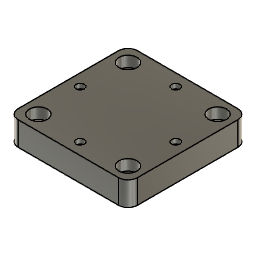
Base_North v3 (Autodesk Fusion 360 design; units mm, degrees)
Autodesk Fusion 360 part; units mm, degrees
note: some values were not read from the file. Set by a fixed rule: which sketch regions a step uses.
sketch "Sketch1" plane through (0, 0, 0) normal (0, 0, 1) x (1, 0, 0)
  line L0 (0, 0) -> (-50, 0)
  line L1 (-50, 0) -> (-50, 50)
  line L2 (-50, 50) -> (0, 50)
  line L3 (0, 50) -> (0, 0)
  dimension "d1" = 50
  dimension "d2" = 50
  constraint horizontal L0
  constraint vertical L1
  constraint horizontal L2
  constraint vertical L3
  constraint coincident L0.start L3.end
  measures "d1" distance of L0.start L0.end
  measures "d2" distance of L0.start L2.end
extrude "Extrude1" add sketch "Sketch1" along normal blind 10
sketch "Sketch2" plane through (0, 0, 10) normal (0, 0, 1) x (-1, 0, 0)
  line L0 (0, -50) -> (50, -50)
  line L1 (50, -50) -> (50, 0)
  line L2 (50, 0) -> (0, 0)
  line L3 (0, 0) -> (0, -50)
  line L4 (50, 0) -> (43.75, 0)
  line L5 (43.75, 0) -> (43.75, -6.25)
  line L6 (43.75, -6.25) -> (50, -6.25)
  line L7 (50, -6.25) -> (50, 0)
  line L8 (50, -50) -> (43.75, -50)
  line L9 (43.75, -50) -> (43.75, -43.75)
  line L10 (43.75, -43.75) -> (50, -43.75)
  line L11 (50, -43.75) -> (50, -50)
  line L12 (0, -50) -> (6.25, -50)
  line L13 (6.25, -50) -> (6.25, -43.75)
  line L14 (6.25, -43.75) -> (0, -43.75)
  line L15 (0, -43.75) -> (0, -50)
  line L16 (0, 0) -> (6.25, 0)
  line L17 (6.25, 0) -> (6.25, -6.25)
  line L18 (6.25, -6.25) -> (0, -6.25)
  line L19 (0, -6.25) -> (0, 0)
  circle A0 centre (43.75, -43.75) radius 3.75
  circle A1 centre (6.25, -43.75) radius 3.75
  circle A2 centre (43.75, -6.25) radius 3.75
  circle A3 centre (6.25, -6.25) radius 3.75
  dimension "d5" = 6.25
  dimension "d6" = 6.25
  dimension "d7" = 6.25
  dimension "d8" = 6.25
  dimension "d9" = 6.25
  dimension "d10" = 6.25
  dimension "d11" = 6.25
  dimension "d12" = 6.25
  dimension "d13" = 7.5
  dimension "d14" = 7.5
  dimension "d15" = 7.5
  dimension "d16" = 7.5
  constraint horizontal L4
  constraint vertical L5
  constraint horizontal L6
  constraint vertical L7
  constraint coincident L1.end L2.start
  constraint horizontal L8
  constraint vertical L9
  constraint horizontal L10
  constraint vertical L11
  constraint coincident L0.end L1.start
  constraint horizontal L12
  constraint vertical L13
  constraint horizontal L14
  constraint vertical L15
  constraint coincident L0.start L3.end
  constraint horizontal L16
  constraint vertical L17
  constraint horizontal L18
  constraint vertical L19
  constraint coincident L2.end L3.start
  constraint coincident L9.end L10.start
  constraint coincident L13.end L14.start
  constraint coincident L5.end L6.start
  constraint coincident L17.end L18.start
  measures "d5" distance of L1.end L4.end
  measures "d6" distance of L1.end L6.end
  measures "d7" distance of L0.end L8.end
  measures "d8" distance of L0.end L10.end
  measures "d9" distance of L0.start L12.end
  measures "d10" distance of L0.start L14.end
  measures "d11" distance of L2.end L16.end
  measures "d12" distance of L2.end L18.end
  measures "d13" diameter of A0
  measures "d14" diameter of A1
  measures "d15" diameter of A2
  measures "d16" diameter of A3
extrude "Extrude2" cut sketch "Sketch2" against normal blind 4.5 contours L13 L14 A1 | L13 L14 A1 | L9 L10 A0 | L9 L10 A0 | L17 L18 A3 | L17 L18 A3 | L5 L6 A2 | L5 L6 A2
sketch "Sketch3" plane through (0, 0, 5.5) normal (0, 0, 1) x (-1, 0, 0)
  circle A0 centre (43.75, -43.75) radius 3.75
  circle A1 centre (43.75, -43.75) radius 2.25
  dimension "d19" = 4.5
  constraint concentric A0 A1
  measures "d19" diameter of A1
extrude "Extrude3" cut sketch "Sketch3" against normal blind 10 contours A1
sketch "Sketch4" plane through (0, 0, 5.5) normal (0, 0, 1) x (-1, 0, 0)
  circle A0 centre (6.25, -43.75) radius 3.75
  circle A1 centre (6.25, -43.75) radius 2.25
  dimension "d22" = 4.5
  constraint concentric A0 A1
  measures "d22" diameter of A1
extrude "Extrude4" cut sketch "Sketch4" against normal blind 10 contours A1
sketch "Sketch5" plane through (0, 0, 5.5) normal (0, 0, 1) x (-1, 0, 0)
  circle A0 centre (43.75, -6.25) radius 3.75
  circle A1 centre (43.75, -6.25) radius 2.25
  dimension "d25" = 4.5
  constraint concentric A0 A1
  measures "d25" diameter of A1
extrude "Extrude5" cut sketch "Sketch5" against normal blind 10 contours A1
sketch "Sketch6" plane through (0, 0, 5.5) normal (0, 0, 1) x (-1, 0, 0)
  circle A0 centre (6.25, -6.25) radius 3.75
  circle A1 centre (6.25, -6.25) radius 2.25
  dimension "d28" = 4.5
  constraint concentric A0 A1
  measures "d28" diameter of A1
extrude "Extrude6" cut sketch "Sketch6" against normal blind 10 contours A1
sketch "Sketch7" plane through (0, 0, 10) normal (0, 0, 1) x (-1, 0, 0)
  circle A0 centre (6.25, -43.75) radius 3.75
  circle A1 centre (6.25, -6.25) radius 3.75
  circle A2 centre (43.75, -43.75) radius 3.75
  circle A3 centre (43.75, -6.25) radius 3.75
  line L0 (0, -50) -> (50, -50)
  line L1 (50, -50) -> (50, 0)
  line L2 (50, 0) -> (0, 0)
  line L3 (0, 0) -> (0, -50)
  line L4 (50, 0) -> (37.5, 0)
  line L5 (37.5, 0) -> (37.5, -12.5)
  line L6 (37.5, -12.5) -> (50, -12.5)
  line L7 (50, -12.5) -> (50, 0)
  line L8 (50, -50) -> (37.5, -50)
  line L9 (37.5, -50) -> (37.5, -37.5)
  line L10 (37.5, -37.5) -> (50, -37.5)
  line L11 (50, -37.5) -> (50, -50)
  line L12 (0, -50) -> (12.5, -50)
  line L13 (12.5, -50) -> (12.5, -37.5)
  line L14 (12.5, -37.5) -> (0, -37.5)
  line L15 (0, -37.5) -> (0, -50)
  line L16 (0, 0) -> (12.5, 0)
  line L17 (12.5, 0) -> (12.5, -12.5)
  line L18 (12.5, -12.5) -> (0, -12.5)
  line L19 (0, -12.5) -> (0, 0)
  line L20 (37.5, -12.5) -> (35.5, -12.5)
  line L21 (35.5, -12.5) -> (35.5, -14.5)
  line L22 (35.5, -14.5) -> (37.5, -14.5)
  line L23 (37.5, -14.5) -> (37.5, -12.5)
  line L24 (37.5, -37.5) -> (35.5, -37.5)
  line L25 (35.5, -37.5) -> (35.5, -35.5)
  line L26 (35.5, -35.5) -> (37.5, -35.5)
  line L27 (37.5, -35.5) -> (37.5, -37.5)
  line L28 (12.5, -37.5) -> (14.5, -37.5)
  line L29 (14.5, -37.5) -> (14.5, -35.5)
  line L30 (14.5, -35.5) -> (12.5, -35.5)
  line L31 (12.5, -35.5) -> (12.5, -37.5)
  line L32 (12.5, -12.5) -> (14.5, -12.5)
  line L33 (14.5, -12.5) -> (14.5, -14.5)
  line L34 (14.5, -14.5) -> (12.5, -14.5)
  line L35 (12.5, -14.5) -> (12.5, -12.5)
  dimension "d31" = 12.5
  dimension "d32" = 12.5
  dimension "d33" = 12.5
  dimension "d34" = 12.5
  dimension "d35" = 12.5
  dimension "d36" = 12.5
  dimension "d37" = 12.5
  dimension "d38" = 12.5
  dimension "d39" = 2
  dimension "d40" = 2
  dimension "d41" = 2
  dimension "d42" = 2
  dimension "d43" = 2
  dimension "d44" = 2
  dimension "d45" = 2
  dimension "d46" = 2
  constraint horizontal L4
  constraint vertical L5
  constraint horizontal L6
  constraint vertical L7
  constraint coincident L1.end L2.start
  constraint horizontal L8
  constraint vertical L9
  constraint horizontal L10
  constraint vertical L11
  constraint coincident L0.end L1.start
  constraint horizontal L12
  constraint vertical L13
  constraint horizontal L14
  constraint vertical L15
  constraint coincident L0.start L3.end
  constraint horizontal L16
  constraint vertical L17
  constraint horizontal L18
  constraint vertical L19
  constraint coincident L2.end L3.start
  constraint horizontal L20
  constraint vertical L21
  constraint horizontal L22
  constraint vertical L23
  constraint horizontal L24
  constraint vertical L25
  constraint horizontal L26
  constraint vertical L27
  constraint horizontal L28
  constraint vertical L29
  constraint horizontal L30
  constraint vertical L31
  constraint horizontal L32
  constraint vertical L33
  constraint horizontal L34
  constraint vertical L35
  measures "d31" distance of L1.end L4.end
  measures "d32" distance of L1.end L6.end
  measures "d33" distance of L0.end L8.end
  measures "d34" distance of L0.end L10.end
  measures "d35" distance of L0.start L12.end
  measures "d36" distance of L0.start L14.end
  measures "d37" distance of L2.end L16.end
  measures "d38" distance of L2.end L18.end
  measures "d39" distance of L5.end L20.end
  measures "d40" distance of L5.end L22.end
  measures "d41" distance of L9.end L24.end
  measures "d42" distance of L9.end L26.end
  measures "d43" distance of L13.end L28.end
  measures "d44" distance of L13.end L30.end
  measures "d45" distance of L17.end L32.end
  measures "d46" distance of L17.end L34.end
extrude "Extrude7" add sketch "Sketch7" along normal blind 2 contours L24 L25 L26 L27 | L20 L21 L22 L23 | L32 L33 L34 L35 | L28 L29 L30 L31
extrude "Extrude8" cut 4 faces at (-13.1667, 36.1667, 12) (-13.1667, 13.1667, 12) (-36.1667, 13.1667, 12) (-36.8333, 36.8333, 12) along direction (0, 0, -1) blind 2
fillet "Fillet1" radius 4 1 edges at (0, 50, 5)
fillet "Fillet2" radius 4 1 edges at (0, 0, 5)
fillet "Fillet3" radius 4 1 edges at (-50, 50, 5)
fillet "Fillet4" radius 4 1 edges at (-50, 0, 5)
sketch "Sketch8" plane through (0, 0, 10) normal (0, 0, 1) x (-1, 0, 0)
  circle A0 centre (6.25, -43.75) radius 3.75
  circle A1 centre (6.25, -6.25) radius 3.75
  circle A2 centre (43.75, -43.75) radius 3.75
  circle A3 centre (43.75, -6.25) radius 3.75
  arc A4 (50, -4) -> (46, 0) centre (46, -4) ccw
  line L0 (46, 0) -> (4, 0)
  arc A5 (4, 0) -> (0, -4) centre (4, -4) ccw
  line L1 (0, -4) -> (0, -46)
  arc A6 (0, -46) -> (4, -50) centre (4, -46) ccw
  line L2 (4, -50) -> (46, -50)
  arc A7 (46, -50) -> (50, -46) centre (46, -46) ccw
  line L3 (50, -46) -> (50, -4)
  line L4 (0, 0) -> (5, 0)
  line L5 (5, 0) -> (5, -5)
  line L6 (5, -5) -> (0, -5)
  line L7 (0, -5) -> (0, 0)
  line L8 (5, -5) -> (45, -5)
  line L9 (45, -5) -> (45, -45)
  line L10 (45, -45) -> (5, -45)
  line L11 (5, -45) -> (5, -5)
  circle A8 centre (25, -45) radius 1.6
  circle A9 centre (45, -25) radius 1.6
  circle A10 centre (25, -5) radius 1.6
  circle A11 centre (5, -25) radius 1.6
  dimension "d59" = 5
  dimension "d60" = 5
  dimension "d61" = 40
  dimension "d62" = 40
  dimension "d63" = 3.2
  dimension "d64" = 3.2
  dimension "d65" = 3.2
  dimension "d66" = 3.2
  constraint horizontal L4
  constraint vertical L5
  constraint horizontal L6
  constraint vertical L7
  constraint coincident L4.start L7.end
  constraint horizontal L8
  constraint vertical L9
  constraint horizontal L10
  constraint vertical L11
  constraint midpoint L10 A8.centre
  constraint midpoint L9 A9.centre
  constraint midpoint L8 A10.centre
  constraint midpoint L11 A11.centre
  measures "d59" distance of L4.start L4.end
  measures "d60" distance of L4.start L6.end
  measures "d61" distance of L5.end L8.end
  measures "d62" distance of L5.end L10.end
  measures "d63" diameter of A8
  measures "d64" diameter of A9
  measures "d65" diameter of A10
  measures "d66" diameter of A11
extrude "Extrude9" cut sketch "Sketch8" against normal blind 2 contours L11 A11 | L11 A11 | L10 A8 | L10 A8 | L9 A9 | L9 A9 | L8 A10 | L8 A10
sketch "Sketch9" plane through (0, 0, 10) normal (0, 0, 1) x (-1, 0, 0)
  circle A0 centre (25, -45) radius 1.6
  circle A1 centre (5, -25) radius 1.6
  circle A2 centre (45, -25) radius 1.6
  circle A3 centre (25, -5) radius 1.6
  circle A4 centre (6.25, -43.75) radius 3.75
  circle A5 centre (6.25, -6.25) radius 3.75
  circle A6 centre (43.75, -43.75) radius 3.75
  circle A7 centre (43.75, -6.25) radius 3.75
  arc A8 (50, -4) -> (46, 0) centre (46, -4) ccw
  line L0 (46, 0) -> (4, 0)
  arc A9 (4, 0) -> (0, -4) centre (4, -4) ccw
  line L1 (0, -4) -> (0, -46)
  arc A10 (0, -46) -> (4, -50) centre (4, -46) ccw
  line L2 (4, -50) -> (46, -50)
  arc A11 (46, -50) -> (50, -46) centre (46, -46) ccw
  line L3 (50, -46) -> (50, -4)
  circle A12 centre (25, -5) radius 1.7
  dimension "d69" = 3.4
  constraint concentric A3 A12
  measures "d69" diameter of A12
extrude "Extrude10" cut sketch "Sketch9" against normal blind 2 contours A12
sketch "Sketch10" plane through (0, 0, 10) normal (0, 0, 1) x (-1, 0, 0)
  circle A0 centre (25, -5) radius 1.7
  circle A1 centre (25, -45) radius 1.6
  circle A2 centre (5, -25) radius 1.6
  circle A3 centre (45, -25) radius 1.6
  circle A4 centre (6.25, -43.75) radius 3.75
  circle A5 centre (6.25, -6.25) radius 3.75
  circle A6 centre (43.75, -43.75) radius 3.75
  circle A7 centre (43.75, -6.25) radius 3.75
  arc A8 (50, -4) -> (46, 0) centre (46, -4) ccw
  line L0 (46, 0) -> (4, 0)
  arc A9 (4, 0) -> (0, -4) centre (4, -4) ccw
  line L1 (0, -4) -> (0, -46)
  arc A10 (0, -46) -> (4, -50) centre (4, -46) ccw
  line L2 (4, -50) -> (46, -50)
  arc A11 (46, -50) -> (50, -46) centre (46, -46) ccw
  line L3 (50, -46) -> (50, -4)
  circle A12 centre (45, -25) radius 1.7
  dimension "d72" = 3.4
  constraint concentric A3 A12
  measures "d72" diameter of A12
extrude "Extrude11" cut sketch "Sketch10" against normal blind 2 contours A12
sketch "Sketch11" plane through (0, 0, 10) normal (0, 0, 1) x (-1, 0, 0)
  circle A0 centre (45, -25) radius 1.7
  circle A1 centre (25, -5) radius 1.7
  circle A2 centre (25, -45) radius 1.6
  circle A3 centre (5, -25) radius 1.6
  circle A4 centre (6.25, -43.75) radius 3.75
  circle A5 centre (6.25, -6.25) radius 3.75
  circle A6 centre (43.75, -43.75) radius 3.75
  circle A7 centre (43.75, -6.25) radius 3.75
  arc A8 (50, -4) -> (46, 0) centre (46, -4) ccw
  line L0 (46, 0) -> (4, 0)
  arc A9 (4, 0) -> (0, -4) centre (4, -4) ccw
  line L1 (0, -4) -> (0, -46)
  arc A10 (0, -46) -> (4, -50) centre (4, -46) ccw
  line L2 (4, -50) -> (46, -50)
  arc A11 (46, -50) -> (50, -46) centre (46, -46) ccw
  line L3 (50, -46) -> (50, -4)
  circle A12 centre (5, -25) radius 1.7
  dimension "d75" = 3.4
  constraint concentric A3 A12
  measures "d75" diameter of A12
extrude "Extrude12" cut sketch "Sketch11" against normal blind 2 contours A12
sketch "Sketch12" plane through (0, 0, 10) normal (0, 0, 1) x (-1, 0, 0)
  circle A0 centre (5, -25) radius 1.7
  circle A1 centre (45, -25) radius 1.7
  circle A2 centre (25, -5) radius 1.7
  circle A3 centre (25, -45) radius 1.6
  circle A4 centre (6.25, -43.75) radius 3.75
  circle A5 centre (6.25, -6.25) radius 3.75
  circle A6 centre (43.75, -43.75) radius 3.75
  circle A7 centre (43.75, -6.25) radius 3.75
  arc A8 (50, -4) -> (46, 0) centre (46, -4) ccw
  line L0 (46, 0) -> (4, 0)
  arc A9 (4, 0) -> (0, -4) centre (4, -4) ccw
  line L1 (0, -4) -> (0, -46)
  arc A10 (0, -46) -> (4, -50) centre (4, -46) ccw
  line L2 (4, -50) -> (46, -50)
  arc A11 (46, -50) -> (50, -46) centre (46, -46) ccw
  line L3 (50, -46) -> (50, -4)
  circle A12 centre (25, -45) radius 1.7
  dimension "d78" = 3.4
  constraint concentric A3 A12
  measures "d78" diameter of A12
extrude "Extrude13" cut sketch "Sketch12" against normal blind 2 contours A12
